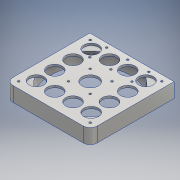
# Autodesk Inventor part: Cup_Dispenser_Stepper_Montage
Saved by Autodesk Inventor 2016 (Build 200138000, 138)
## iProperties
Created: 2015-07-09
Part Number: Cup_Dispenser_Stepper_Montage
Material: Generic
Document SubType Name: Modeling
Designer: marku
Density: 1 g/cm^3
Appearance: Aluminum - Flat
Author: marku
Autodesk Inventor part; units mm, degrees
ref_plane "YZ Plane" through (0, 0, 0) normal (1, 0, 0) x (0, 1, 0)
ref_plane "XZ Plane" through (0, 0, 0) normal (0, 1, 0) x (-1, 0, 0)
ref_plane "XY Plane" through (0, 0, 0) normal (0, 0, 1) x (1, 0, 0)
sketch "Sketch1" plane through (0, 0, 0) normal (0, 0, 1) x (1, 0, 0)
  circle A0 centre (-51, -113.7922) radius 1.5 projected
  circle A1 centre (51, -113.7922) radius 1.5 projected
  circle A2 centre (-51, 108.2078) radius 1.5 projected
  circle A3 centre (51, 6.2078) radius 1.5 projected
  circle A4 centre (51, 108.2078) radius 1.5 projected
  circle A5 centre (-51, 6.2078) radius 1.5 projected
  circle A6 centre (51, -11.7922) radius 1.5 projected
  circle A7 centre (-51, -11.7922) radius 1.5 projected
  circle A8 centre (0, -62.7922) radius 57 projected
  circle A9 centre (0, 57.2078) radius 57 projected
  line L0 (-60, 117.2078) -> (-60, -112.7922) projected
  arc A10 (-60, -112.7922) -> (-50, -122.7922) centre (-50, -112.7922) ccw projected
  line L1 (-50, -122.7922) -> (50, -122.7922) projected
  arc A11 (50, -122.7922) -> (60, -112.7922) centre (50, -112.7922) ccw projected
  line L2 (60, -112.7922) -> (60, 117.2078) projected
  line L3 (60, 117.2078) -> (-60, 117.2078) projected
  line L4 (-60, -2.7922) -> (60, -2.7922) projected
  point P0 (0, 0)
extrude "Extrusion1" add sketch "Sketch1" along normal blind 18 contours L4 L2 A11 L1 A10 L0
sketch "Sketch2" plane through (0, 0, 18) normal (0, 0, 1) x (1, 0, 0)
  circle A0 centre (0, -62.7922) radius 57 projected
  circle A1 centre (-51, -11.7922) radius 1.5 projected
  circle A2 centre (51, -11.7922) radius 1.5 projected
  circle A3 centre (51, -113.7922) radius 1.5 projected
  circle A4 centre (-51, -113.7922) radius 1.5 projected
  arc A5 (-60, -112.7922) -> (-50, -122.7922) centre (-50, -112.7922) ccw projected
  line L0 (-50, -122.7922) -> (50, -122.7922) projected
  arc A6 (50, -122.7922) -> (60, -112.7922) centre (50, -112.7922) ccw projected
  line L1 (60, -112.7922) -> (60, -2.7922) projected
  line L2 (60, -2.7922) -> (-60, -2.7922) projected
  line L3 (-60, -2.7922) -> (-60, -112.7922) projected
  point P0 (0, 0)
extrude "Extrusion2" add sketch "Sketch2" along normal blind 3 contours A0 | L3 L2 L1 A6 L0 A5
sketch "Sketch3" plane through (0, 0, 21) normal (0, 0, 1) x (1, 0, 0)
  circle A0 centre (0, -62.7922) radius 57 projected
  circle A1 centre (0, -62.7922) radius 11.5
  point P0 (0, 0)
  dimension "d4" = 23
  constraints: 1 centre point, 1 coincident
  measures "d4" diameter of A1
extrude "Extrusion3" cut sketch "Sketch3" against normal up to next contours A1
sketch "Sketch4" plane through (0, 0, 21) normal (0, 0, 1) x (1, 0, 0)
  circle A0 centre (0, -62.7922) radius 11.5 construction
  line L0 (-15.5, -47.2922) -> (15.5, -47.2922) construction
  line L1 (15.5, -47.2922) -> (15.5, -78.2922) construction
  line L2 (15.5, -78.2922) -> (-15.5, -78.2922) construction
  line L3 (-15.5, -78.2922) -> (-15.5, -47.2922) construction
  line L4 (-15.5, -47.2922) -> (15.5, -78.2922) construction
  line L5 (15.5, -47.2922) -> (-15.5, -78.2922) construction
  point P0 (0, 0)
  dimension "d7" = 31
  dimension "d8" = 31
  constraints: 12 end point, 4 coincident, 2 midpoint, 2 parallel, 1 horizontal, 1 perpendicular
  measures "d7" distance of L1.end L2.end
  measures "d8" distance of L0.end L1.end
hole "Hole1" at (15.5, -78.2922, 21) at (-15.5, -78.2922, 21) at (-15.5, -47.2922, 21) at (15.5, -47.2922, 21) direction (0, 0, -1) diameter 3 depth 8 tip angle 118
thicken "Thicken1" operation add thickness 0.6 both sides no extend neighbours yes toward (0, -1, 0) faces at (20, -2.7922, 7)
sketch "Sketch5" plane through (0, 0, 21) normal (0, 0, 1) x (1, 0, 0)
  line L0 (0, -62.7922) -> (0, -173.9711) construction
  line L1 (-30, -9.3922) -> (30, -9.3922)
  line L2 (30, -9.3922) -> (30, -33.3922)
  line L3 (30, -33.3922) -> (-30, -33.3922)
  line L4 (-30, -33.3922) -> (-30, -9.3922)
  line L5 (-30, -9.3922) -> (30, -33.3922) construction
  line L6 (30, -9.3922) -> (-30, -33.3922) construction
  line L7 (60, -3.3922) -> (-60, -3.3922) projected
  point P0 (0, -21.3922)
  point P1 (0, -9.3922)
  point P2 (0, -33.3922)
  dimension "d21" = 60
  dimension "d22" = 24
  dimension "d23" = 6
  constraints: 14 end point, 4 coincident, 4 midpoint, 2 parallel, 1 horizontal, 1 perpendicular, 1 vertical, 1 other
  measures "d21" distance of L2.end L3.end
  measures "d22" distance of L1.end L2.end
  measures "d23" distance from line of L7 L1.start
hole "Hole2" at (30, -9.3922, 21) at (30, -33.3922, 21) at (0, -9.3922, 21) at (0, -33.3922, 21) at (-30, -33.3922, 21) at (-30, -9.3922, 21) direction (0, 0, -1) diameter 3 depth 2 tip angle 118
sketch "Sketch6" plane through (0, 0, 21) normal (0, 0, 1) x (1, 0, 0)
  circle A0 centre (-30, -33.3922) radius 1.5 projected
  circle A1 centre (0, -9.3922) radius 1.5 projected
  circle A2 centre (30, -9.3922) radius 1.5 projected
  circle A3 centre (30, -33.3922) radius 1.5 projected
  circle A4 centre (0, -33.3922) radius 1.5 projected
  circle A5 centre (-30, -9.3922) radius 1.5 projected
  circle A6 centre (-15.5, -47.2922) radius 1.5 projected
  circle A7 centre (15.5, -78.2922) radius 1.5 projected
  circle A8 centre (-15.5, -78.2922) radius 1.5 projected
  circle A9 centre (15.5, -47.2922) radius 1.5 projected
  circle A10 centre (0, -62.7922) radius 11.5 projected
  circle A11 centre (-51, -113.7922) radius 1.5 projected
  circle A12 centre (51, -113.7922) radius 1.5 projected
  circle A13 centre (51, -11.7922) radius 1.5 projected
  circle A14 centre (-51, -11.7922) radius 1.5 projected
  arc A15 (-60, -112.7922) -> (-50, -122.7922) centre (-50, -112.7922) ccw projected
  line L0 (-50, -122.7922) -> (50, -122.7922) projected
  arc A16 (50, -122.7922) -> (60, -112.7922) centre (50, -112.7922) ccw projected
  line L1 (60, -112.7922) -> (60, -3.3922) projected
  line L2 (60, -3.3922) -> (-60, -3.3922) projected
  line L3 (-60, -3.3922) -> (-60, -112.7922) projected
  line L4 (0, 0) -> (0, -151.5305) construction
  circle A17 centre (39, -22.2922) radius 10.5
  circle A18 centre (39, -48.2922) radius 10.5
  circle A19 centre (39, -74.2922) radius 10.5
  circle A20 centre (39, -100.2922) radius 10.5
  circle A21 centre (13, -100.2922) radius 10.5
  circle A22 centre (13, -22.2922) radius 10.5
  circle A23 centre (-39, -22.2922) radius 10.5
  circle A24 centre (-39, -48.2922) radius 10.5
  circle A25 centre (-39, -74.2922) radius 10.5
  circle A26 centre (-39, -100.2922) radius 10.5
  circle A27 centre (-13, -100.2922) radius 10.5
  circle A28 centre (-13, -22.2922) radius 10.5
  dimension "d32" = 21
  dimension "d39" = 26
  dimension "d46" = 26
  dimension "d53" = 26
  dimension "d59" = 26
  constraints: 12 centre point, 6 symmetric about line, 2 end point, 2 horizontal, 2 vertical, 16 other
  measures "d32" diameter of A17
  measures "d39" distance of A17.centre A18.centre
  measures "d46" distance of A20.centre A21.centre
  measures "d53" distance of A17.centre A22.centre
  measures "d59" distance of A28.centre A22.centre
extrude "Extrusion4" cut sketch "Sketch6" against normal up to surface (3 mm away) contours A17 | A18 | A19 | A20 | A21 | A22 | A23 | A24 | A25 | A26 | A27 | A28
equation "\"d0\" = 6 * thickness"
equation "\"d2\" = thickness"
equation "\"d5\" = thickness"
equation "\"d29\" = 0.666667 * thickness"
equation "\"thickness\" = 3"
body "Solid1"
